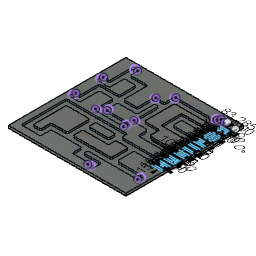
maze-v14 (Autodesk Fusion 360 design; units mm, degrees)
Autodesk Fusion 360 part; units mm, degrees
sketch "Sketch1" plane through (0, 0, 0) normal (0, 0, 1) x (1, 0, 0)
  line L0 (0, 0) -> (1000, 0)
  line L1 (1000, 0) -> (1000, 1000)
  line L2 (1000, 1000) -> (0, 1000)
  line L3 (0, 1000) -> (0, 0)
  dimension "d1" = 1000
  dimension "d2" = 1000
  constraint horizontal L0
  constraint vertical L1
  constraint horizontal L2
  constraint vertical L3
  constraint coincident L0.start L3.end
  measures "d1" distance of L0.start L2.end
  measures "d2" distance of L0.start L0.end
extrude "Extrude1" add sketch "Sketch1" along normal blind 21
sketch "top" plane through (0, 0, 21) normal (0, 0, 1) x (-1, 0, 0)
  line L0 (0, -1000) -> (0, 0)
  line L1 (0, 0) -> (-1000, 0)
  line L2 (-1000, 0) -> (-1000, -1000)
  line L3 (-1000, -1000) -> (0, -1000)
  arc A0 (-525, -126.8622) -> (-535, -116.8622) centre (-535, -126.8622) ccw
  arc A1 (-559.9586, -282.9891) -> (-569.9586, -292.9891) centre (-559.9586, -292.9891) ccw
  arc A2 (-535, -150) -> (-525, -140) centre (-535, -140) ccw
  line L4 (-300, -620.3885) -> (-300, -540)
  line L5 (-525, -140) -> (-525, -126.8622)
  arc A3 (-519.9586, -383.45) -> (-509.9586, -393.45) centre (-509.9586, -383.45) ccw
  arc A4 (-360, -282.9891) -> (-350, -272.9891) centre (-360, -272.9891) ccw
  arc A5 (-475, -140) -> (-465, -150) centre (-465, -140) ccw
  arc A6 (-579.9586, -344.6286) -> (-569.9586, -334.6286) centre (-579.9586, -334.6286) ccw
  line L6 (-569.9586, -404.6286) -> (-569.9586, -433.45)
  line L7 (-300, -332.9891) -> (-300, -383.45)
  line L8 (-300, -210) -> (-300, -283.8474)
  arc A7 (-360, -393.45) -> (-350, -383.45) centre (-360, -383.45) ccw
  arc A8 (-300, -383.45) -> (-290, -393.45) centre (-290, -383.45) ccw
  line L9 (-569.9586, -292.9891) -> (-569.9586, -334.6286)
  line L10 (-509.9586, -332.9891) -> (-360, -332.9891)
  line L11 (-519.9586, -383.45) -> (-519.9586, -342.9891)
  line L12 (-475, -200) -> (-360, -200)
  line L13 (-350, -210) -> (-350, -272.9891)
  line L14 (-890, -344.6286) -> (-735, -344.6286)
  arc A9 (-92.3471, -692.4262) -> (-82.3471, -682.4262) centre (-92.3471, -682.4262) ccw
  arc A10 (-660, -824.2821) -> (-650, -814.2821) centre (-660, -814.2821) ccw
  line L15 (-677.1097, -535) -> (-677.1097, -599.6568)
  line L16 (-700, -764.2821) -> (-700, -709.2787)
  arc A11 (-150, -897.4685) -> (-160, -887.4685) centre (-160, -897.4685) ccw
  line L17 (-300, -690.3885) -> (-300, -877.4685)
  arc A12 (-625, -56.8622) -> (-615, -66.8622) centre (-615, -56.8622) ccw
  arc A13 (-300, -877.4685) -> (-290, -887.4685) centre (-290, -877.4685) ccw
  arc A14 (-700, -709.2787) -> (-710, -699.2787) centre (-710, -709.2787) ccw
  line L18 (-132.3471, -632.4262) -> (-132.3471, -485.0006)
  line L19 (-840, -394.6286) -> (-715.6967, -394.6286)
  line L20 (-415.2274, -820.725) -> (-415.2274, -690.3885)
  arc A15 (-710, -774.2821) -> (-700, -764.2821) centre (-710, -764.2821) ccw
  line L21 (-465.2274, -770.725) -> (-465.2274, -640.3885)
  line L22 (-82.3471, -682.4262) -> (-82.3471, -525)
  arc A16 (-840, -824.2821) -> (-850, -834.2821) centre (-840, -834.2821) ccw
  line L23 (-250, -632.4262) -> (-250, -490)
  line L24 (-850, -639.2787) -> (-850, -535)
  line L25 (-497.671, -569.6568) -> (-497.671, -770.725)
  line L26 (-100, -837.4685) -> (-100, -770)
  arc A17 (-650, -659.2787) -> (-660, -649.2787) centre (-660, -659.2787) ccw
  arc A18 (-160, -837.4685) -> (-150, -827.4685) centre (-160, -827.4685) ccw
  line L27 (-290, -887.4685) -> (-160, -887.4685)
  arc A19 (-250, -632.4262) -> (-240, -642.4262) centre (-240, -632.4262) ccw
  arc A20 (-677.1097, -599.6568) -> (-667.1097, -609.6568) centre (-667.1097, -599.6568) ccw
  line L28 (-675, -334.6286) -> (-675, -210)
  line L29 (-900, -940) -> (-900, -784.2821)
  arc A21 (-627.1097, -549.6568) -> (-617.1097, -559.6568) centre (-617.1097, -549.6568) ccw
  arc A22 (-890, -774.2821) -> (-900, -784.2821) centre (-890, -784.2821) ccw
  line L30 (-715.6967, -394.6286) -> (-579.9586, -394.6286)
  arc A23 (-850, -465) -> (-840, -475) centre (-840, -465) ccw
  line L31 (-625, -50) -> (-625, -56.8622)
  line L32 (-240, -642.4262) -> (-142.3471, -642.4262)
  line L33 (-100, -837.4685) -> (-100, -950)
  arc A24 (-405.2274, -680.3885) -> (-415.2274, -690.3885) centre (-405.2274, -690.3885) ccw
  arc A25 (-725, -210) -> (-735, -200) centre (-735, -210) ccw
  line L34 (-650, -814.2821) -> (-650, -659.2787)
  line L35 (-547.671, -830.725) -> (-547.671, -857.0303)
  arc A26 (-475.2274, -780.725) -> (-465.2274, -770.725) centre (-475.2274, -770.725) ccw
  arc A27 (-677.1097, -535) -> (-687.1097, -525) centre (-687.1097, -535) ccw
  arc A28 (-140, -710.014) -> (-150, -720.014) centre (-140, -720.014) ccw
  arc A29 (-240, -692.4262) -> (-250, -702.4262) centre (-240, -702.4262) ccw
  line L36 (-650, -774.2821) -> (-649.9827, -774.2821)
  arc A30 (-675, -106.8622) -> (-665, -116.8622) centre (-665, -106.8622) ccw
  line L37 (-487.671, -830.725) -> (-425.2274, -830.725)
  line L38 (-547.671, -619.6568) -> (-547.671, -830.725)
  arc A31 (-455.2274, -630.3885) -> (-465.2274, -640.3885) centre (-455.2274, -640.3885) ccw
  line L39 (-497.671, -840.725) -> (-497.671, -907.0303)
  line L40 (-890, -774.2821) -> (-710, -774.2821)
  arc A32 (-840, -394.6286) -> (-850, -404.6286) centre (-840, -404.6286) ccw
  arc A33 (-675, -334.6286) -> (-665, -344.6286) centre (-665, -334.6286) ccw
  arc A34 (-840, -525) -> (-850, -535) centre (-840, -535) ccw
  line L41 (-627.1097, -485) -> (-627.1097, -549.6568)
  line L42 (-725, -334.6286) -> (-725, -210)
  line L43 (-675, -106.8622) -> (-675, -50)
  line L44 (-840, -475) -> (-637.1097, -475)
  line L45 (-850, -940) -> (-850, -927.0303)
  line L46 (-850, -857.0303) -> (-850, -834.2821)
  line L47 (-665, -344.6286) -> (-579.9586, -344.6286)
  line L48 (-900, -689.2787) -> (-900, -475)
  arc A35 (-735, -344.6286) -> (-725, -334.6286) centre (-735, -334.6286) ccw
  line L49 (-840, -525) -> (-687.1097, -525)
  line L50 (-840, -824.2821) -> (-660, -824.2821)
  line L51 (-675, -150) -> (-950, -150)
  line L52 (-660, -649.2787) -> (-840, -649.2787)
  arc A36 (-665, -200) -> (-675, -210) centre (-665, -210) ccw
  arc A37 (-900, -689.2787) -> (-890, -699.2787) centre (-890, -689.2787) ccw
  arc A38 (-142.3471, -642.4262) -> (-132.3471, -632.4262) centre (-142.3471, -632.4262) ccw
  arc A39 (-627.1097, -485) -> (-637.1097, -475) centre (-637.1097, -485) ccw
  line L53 (-710, -699.2787) -> (-890, -699.2787)
  arc A40 (-850, -639.2787) -> (-840, -649.2787) centre (-840, -639.2787) ccw
  arc A41 (-850, -857.0303) -> (-840, -867.0303) centre (-840, -857.0303) ccw
  arc A42 (-475, -76.8622) -> (-485, -66.8622) centre (-485, -76.8622) ccw
  line L54 (-350, -342.9891) -> (-350, -383.45)
  arc A43 (-569.9586, -433.45) -> (-559.9586, -443.45) centre (-559.9586, -433.45) ccw
  line L55 (-360, -393.45) -> (-509.9586, -393.45)
  line L56 (-300, -332.9891) -> (-300, -283.8474)
  line L57 (-465, -150) -> (-300, -150)
  arc A44 (-350, -342.9891) -> (-360, -332.9891) centre (-360, -342.9891) ccw
  line L58 (-500, -530) -> (-310, -530)
  arc A45 (-509.9586, -332.9891) -> (-519.9586, -342.9891) centre (-509.9586, -342.9891) ccw
  arc A46 (-350, -210) -> (-360, -200) centre (-360, -210) ccw
  line L59 (-360, -282.9891) -> (-559.9586, -282.9891)
  line L60 (-475, -76.8622) -> (-475, -140)
  arc A47 (-290, -200) -> (-300, -210) centre (-290, -210) ccw
  line L61 (-154.4283, -108.8474) -> (-110, -108.8474)
  arc A48 (-204.4283, -58.8474) -> (-214.4283, -68.8474) centre (-204.4283, -68.8474) ccw
  line L62 (-214.4283, -140) -> (-214.4283, -68.8474)
  arc A49 (-60, -443.45) -> (-50, -433.45) centre (-60, -433.45) ccw
  arc A50 (-110, -393.45) -> (-100, -383.45) centre (-110, -383.45) ccw
  arc A51 (-224.4283, -150) -> (-214.4283, -140) centre (-224.4283, -140) ccw
  line L63 (-164.4283, -190) -> (-164.4283, -118.8474)
  line L64 (-557.671, -867.0303) -> (-840, -867.0303)
  arc A52 (-100, -118.8474) -> (-110, -108.8474) centre (-110, -118.8474) ccw
  arc A53 (-154.4283, -108.8474) -> (-164.4283, -118.8474) centre (-154.4283, -118.8474) ccw
  arc A54 (-122.3471, -475.0006) -> (-132.3471, -485.0006) centre (-122.3471, -485.0006) ccw
  arc A55 (-174.4283, -200) -> (-164.4283, -190) centre (-174.4283, -190) ccw
  line L65 (-50, -68.8474) -> (-50, -316.2628)
  arc A56 (-50, -68.8474) -> (-60, -58.8474) centre (-60, -68.8474) ccw
  line L66 (-50, -316.2628) -> (-50, -433.45)
  line L67 (-204.4283, -58.8474) -> (-60, -58.8474)
  line L68 (-100, -118.8474) -> (-100, -383.45)
  line L69 (-617.1097, -559.6568) -> (-507.671, -559.6568)
  line L70 (-507.671, -917.0303) -> (-840, -917.0303)
  line L71 (-615, -66.8622) -> (-485, -66.8622)
  arc A57 (-569.9586, -404.6286) -> (-579.9586, -394.6286) centre (-579.9586, -404.6286) ccw
  line L72 (-140, -710.014) -> (-49.1705, -710.014)
  line L73 (-535, -116.8622) -> (-665, -116.8622)
  line L74 (-500, -480) -> (-260, -480)
  line L75 (-110, -393.45) -> (-290, -393.45)
  line L76 (-300, -150) -> (-224.4283, -150)
  line L77 (-240, -692.4262) -> (-92.3471, -692.4262)
  line L78 (-290, -200) -> (-174.4283, -200)
  line L79 (-60, -443.45) -> (-559.9586, -443.45)
  line L80 (-675, -150) -> (-535, -150)
  line L81 (-667.1097, -609.6568) -> (-557.671, -609.6568)
  arc A58 (-300, -690.3885) -> (-310, -680.3885) centre (-310, -690.3885) ccw
  line L82 (0, 0) -> (-1000, 0)
  arc A59 (-557.671, -867.0303) -> (-547.671, -857.0303) centre (-557.671, -857.0303) ccw
  line L83 (-850, -465) -> (-850, -404.6286)
  arc A60 (-310, -630.3885) -> (-300, -620.3885) centre (-310, -620.3885) ccw
  arc A61 (-497.671, -770.725) -> (-487.671, -780.725) centre (-487.671, -770.725) ccw
  line L84 (-250, -702.4262) -> (-250, -827.4685)
  line L85 (-665, -200) -> (-475, -200)
  line L86 (-405.2274, -680.3885) -> (-310, -680.3885)
  line L87 (-1000, 0) -> (-1000, -1000)
  line L88 (-900, -475) -> (-900, -354.6286)
  line L89 (-150, -897.4685) -> (-150, -950)
  line L90 (-150, -827.4685) -> (-150, -720.014)
  line L91 (-1000, -1000) -> (0, -1000)
  line L92 (-455.2274, -630.3885) -> (-310, -630.3885)
  arc A62 (-487.671, -830.725) -> (-497.671, -840.725) centre (-487.671, -840.725) ccw
  line L93 (-240, -837.4685) -> (-160, -837.4685)
  line L94 (-487.671, -780.725) -> (-475.2274, -780.725)
  line L95 (-0.0099, -1000) -> (-0.0018, 0)
  arc A63 (-250, -827.4685) -> (-240, -837.4685) centre (-240, -827.4685) ccw
  arc A64 (-890, -344.6286) -> (-900, -354.6286) centre (-890, -354.6286) ccw
  line L96 (-90, -760) -> (-50.0078, -760)
  arc A65 (-90, -760) -> (-100, -770) centre (-90, -770) ccw
  line L97 (-735, -200) -> (-950, -200)
  line L98 (-122.3471, -475.0006) -> (-49.8349, -475.0006)
  line L99 (-0.0056, -475.0006) -> (0, -475.0006)
  line L100 (-82.3471, -525) -> (-50.0058, -525)
  line L101 (-860, -950) -> (-890, -950)
  arc A66 (-250, -490) -> (-260, -480) centre (-260, -490) ccw
  arc A67 (-300, -540) -> (-310, -530) centre (-310, -540) ccw
  arc A68 (-425.2274, -830.725) -> (-415.2274, -820.725) centre (-425.2274, -820.725) ccw
  arc A69 (-497.671, -569.6568) -> (-507.671, -559.6568) centre (-507.671, -569.6568) ccw
  arc A70 (-547.671, -619.6568) -> (-557.671, -609.6568) centre (-557.671, -619.6568) ccw
  arc A71 (-507.671, -917.0303) -> (-497.671, -907.0303) centre (-507.671, -907.0303) ccw
  arc A72 (-840, -917.0303) -> (-850, -927.0303) centre (-840, -927.0303) ccw
  arc A73 (-860, -950) -> (-850, -940) centre (-860, -940) ccw
  arc A74 (-900, -940) -> (-890, -950) centre (-890, -940) ccw
  arc A75 (-950, -150) -> (-950, -200) centre (-950, -175) ccw
  arc A76 (-625, -50) -> (-675, -50) centre (-650, -50) ccw
  arc A77 (-50.0058, -525) -> (-50.1768, -475.0006) centre (-50.0058, -500) ccw
  arc A78 (-50.0078, -760) -> (-50.845, -710.014) centre (-50.0078, -735) ccw
  arc A79 (-150, -950) -> (-100, -950) centre (-125, -950) ccw
  arc A80 (-500, -480) -> (-500, -530) centre (-500, -505) ccw
  point P0 (-1000, -1000)
  dimension "d67" = 50
  dimension "d68" = 50
  dimension "d69" = 90
  dimension "d70" = 50
  dimension "d71" = 50
  dimension "d72" = 50
  dimension "d73" = 50
  dimension "d74" = 50
  dimension "d75" = 50
  dimension "d76" = 50
  dimension "d77" = 50
  dimension "d78" = 50
  dimension "d79" = 50
  dimension "d81" = 50
  dimension "d83" = 50
  dimension "d84" = 50
  dimension "d85" = 50
  dimension "d86" = 50
  dimension "d87" = 50
  dimension "d88" = 50
  dimension "d89" = 50
  dimension "d90" = 50
  dimension "d91" = 50
  dimension "d93" = 50
  dimension "d94" = 50
  dimension "d95" = 50
  dimension "d96" = 50
  dimension "d97" = 50
  dimension "d98" = 50
  dimension "d99" = 50
  dimension "d100" = 50
  dimension "d101" = 50
  dimension "d102" = 50
  dimension "d103" = 50
  dimension "d104" = 50
  dimension "d105" = 50
  dimension "d106" = 50
  dimension "d107" = 10
  dimension "d108" = 10
  dimension "d109" = 50
  dimension "d110" = 10
  dimension "d111" = 50
  dimension "d112" = 50
  dimension "d113" = 50
  dimension "d114" = 50
  dimension "d115" = 50
  dimension "d116" = 50
  dimension "d117" = 50
  dimension "d118" = 50
  dimension "d119" = 50
  dimension "d120" = 50
  dimension "d123" = 10
  dimension "d125" = 90
  dimension "d126" = 10
  dimension "d128" = 90
  dimension "d131" = 50
  dimension "d185" = 10
  dimension "d186" = 10
  constraint vertical L45
  constraint perpendicular L45 L50
  constraint perpendicular L34 L50
  constraint perpendicular L34 L52
  constraint perpendicular L24 L52
  constraint perpendicular L24 L49
  constraint perpendicular L15 L49
  constraint perpendicular L15 L81
  constraint perpendicular L38 L81
  constraint perpendicular L15 L37
  constraint perpendicular L20 L81
  constraint perpendicular L20 L86
  constraint perpendicular L23 L86
  constraint vertical L29
  constraint perpendicular L16 L53
  constraint coincident L36.start L34
  constraint collinear L36 L40
  constraint perpendicular L48 L53
  constraint perpendicular L44 L48
  constraint perpendicular L41 L53
  constraint perpendicular L41 L69
  constraint perpendicular L25 L69
  constraint perpendicular L41 L94
  constraint perpendicular L21 L69
  constraint perpendicular L41 L92
  constraint perpendicular L4 L92
  constraint tangent L58 A80
  constraint perpendicular L4 L58
  constraint tangent L74 A80
  constraint horizontal L74
  constraint perpendicular L44 L88
  constraint perpendicular L14 L88
  constraint perpendicular L14 L42
  constraint perpendicular L44 L83
  constraint perpendicular L19 L24
  constraint perpendicular L28 L44
  constraint perpendicular L24 L51
  constraint perpendicular L84 L86
  constraint perpendicular L84 L93
  constraint perpendicular L33 L86
  constraint perpendicular L17 L86
  constraint perpendicular L17 L27
  constraint perpendicular L27 L89
  constraint perpendicular L23 L32
  constraint perpendicular L18 L32
  constraint perpendicular L23 L77
  constraint perpendicular L22 L77
  constraint perpendicular L18 L98
  constraint perpendicular L26 L93
  constraint perpendicular L90 L93
  constraint perpendicular L72 L90
  constraint perpendicular L37 L39
  constraint perpendicular L45 L70
  constraint perpendicular L35 L37
  constraint perpendicular L45 L64
  constraint perpendicular L28 L80
  constraint perpendicular L5 L80
  constraint perpendicular L28 L73
  constraint perpendicular L43 L73
  constraint perpendicular L31 L73
  constraint perpendicular L31 L71
  constraint perpendicular L28 L85
  constraint perpendicular L57 L60
  constraint perpendicular L8 L57
  constraint perpendicular L12 L60
  constraint perpendicular L12 L13
  constraint perpendicular L13 L59
  constraint perpendicular L9 L12
  constraint perpendicular L10 L11
  constraint perpendicular L10 L56
  constraint perpendicular L8 L76
  constraint perpendicular L57 L62
  constraint perpendicular L62 L67
  constraint perpendicular L57 L65
  constraint perpendicular L8 L78
  constraint perpendicular L63 L78
  constraint perpendicular L61 L63
  constraint perpendicular L61 L68
  constraint vertical L68
  constraint parallel L65 L66
  constraint perpendicular L68 L75
  constraint perpendicular L66 L79
  constraint vertical L11
  constraint collinear L45 L46
  constraint perpendicular L54 L75
  constraint perpendicular L7 L75
  constraint collinear L55 L75
  constraint perpendicular L9 L47
  constraint perpendicular L9 L30
  constraint collinear L6 L9
  constraint tangent A12 L31
  constraint tangent A12 L71
  constraint tangent A30 L73
  constraint tangent A30 L43
  constraint equal A12 A30
  constraint tangent A0 L5
  constraint tangent A0 L73
  constraint equal A0 A12
  constraint tangent A42 L71
  constraint tangent A42 L60
  constraint tangent A5 L57
  constraint tangent A5 L60
  constraint equal A5 A42
  constraint tangent A2 L80
  constraint tangent A2 L5
  constraint equal A2 A42
  constraint tangent A36 L85
  constraint tangent L28 A36
  constraint tangent A25 L42
  constraint equal A25 A36
  constraint tangent L14 A35
  constraint tangent L42 A35
  constraint equal A35 A36
  constraint tangent A33 L47
  constraint tangent L28 A33
  constraint equal A33 A36
  constraint tangent A32 L83
  constraint tangent L19 A32
  constraint equal A32 A36
  constraint tangent A23 L83
  constraint tangent A23 L44
  constraint equal A23 A36
  constraint tangent L44 A39
  constraint tangent L41 A39
  constraint equal A36 A39
  constraint tangent A21 L41
  constraint tangent A21 L69
  constraint equal A21 A36
  constraint tangent A27 L49
  constraint tangent L15 A27
  constraint equal A27 A36
  constraint tangent L15 A20
  constraint tangent A20 L81
  constraint equal A20 A36
  constraint tangent L24 A34
  constraint tangent A34 L49
  constraint equal A34 A36
  constraint tangent L52 A40
  constraint tangent L24 A40
  constraint equal A36 A40
  constraint tangent A37 L53
  constraint tangent L48 A37
  constraint equal A36 A37
  constraint tangent A17 L34
  constraint tangent A17 L52
  constraint equal A17 A36
  constraint tangent L16 A14
  constraint tangent A14 L53
  constraint equal A14 A36
  constraint tangent L16 A15
  constraint tangent A15 L40
  constraint equal A15 A36
  constraint tangent A16 L50
  constraint tangent A16 L46
  constraint equal A16 A36
  constraint tangent L29 A22
  constraint tangent A22 L40
  constraint equal A22 A36
  constraint tangent A41 L64
  constraint tangent L46 A41
  constraint equal A36 A41
  constraint tangent L35 A59
  constraint tangent L64 A59
  constraint equal A36 A59
  constraint tangent L39 A62
  constraint tangent L37 A62
  constraint equal A36 A62
  constraint tangent L25 A61
  constraint tangent A61 L94
  constraint equal A36 A61
  constraint tangent A26 L94
  constraint tangent L21 A26
  constraint equal A26 A36
  constraint tangent L20 A24
  constraint tangent A24 L86
  constraint equal A24 A36
  constraint tangent L21 A31
  constraint tangent A31 L92
  constraint equal A31 A36
  constraint tangent L17 A58
  constraint tangent A58 L86
  constraint equal A36 A58
  constraint tangent A60 L92
  constraint tangent L4 A60
  constraint equal A36 A60
  constraint tangent A19 L32
  constraint tangent L23 A19
  constraint equal A19 A36
  constraint tangent A29 L84
  constraint tangent A29 L77
  constraint equal A29 A36
  constraint tangent A9 L77
  constraint tangent A9 L22
  constraint equal A9 A36
  constraint tangent L32 A38
  constraint tangent L18 A38
  constraint equal A36 A38
  constraint tangent L84 A63
  constraint tangent L93 A63
  constraint equal A36 A63
  constraint tangent L17 A13
  constraint tangent A13 L27
  constraint equal A13 A36
  constraint tangent A18 L90
  constraint tangent A18 L93
  constraint equal A18 A36
  constraint tangent A11 L27
  constraint tangent A11 L89
  constraint equal A11 A36
  constraint tangent A28 L90
  constraint tangent A28 L72
  constraint equal A28 A36
  constraint tangent L18 A54
  constraint tangent A54 L98
  constraint equal A36 A54
  constraint tangent A49 L66
  constraint tangent A49 L79
  constraint equal A36 A49
  constraint tangent A50 L68
  constraint tangent A50 L75
  constraint equal A36 A50
  constraint tangent L7 A8
  constraint tangent A8 L75
  constraint equal A8 A36
  constraint tangent A7 L54
  constraint tangent A7 L55
  constraint equal A7 A36
  constraint tangent L54 A44
  constraint tangent L10 A44
  constraint equal A36 A44
  constraint tangent A4 L13
  constraint tangent A4 L59
  constraint equal A4 A36
  constraint tangent L12 A46
  constraint tangent L13 A46
  constraint equal A36 A46
  constraint tangent A47 L78
  constraint tangent L8 A47
  constraint equal A36 A47
  constraint tangent A55 L78
  constraint tangent L63 A55
  constraint equal A36 A55
  constraint tangent L63 A53
  constraint tangent L61 A53
  constraint equal A36 A53
  constraint tangent A48 L62
  constraint tangent A48 L67
  constraint equal A36 A48
  constraint tangent L61 A52
  constraint tangent A52 L68
  constraint equal A36 A52
  constraint tangent A56 L67
  constraint tangent L65 A56
  constraint equal A36 A56
  constraint tangent L11 A45
  constraint tangent L10 A45
  constraint equal A36 A45
  constraint tangent A3 L11
  constraint tangent A3 L55
  constraint equal A3 A36
  constraint tangent L30 A57
  constraint tangent L6 A57
  constraint equal A36 A57
  constraint tangent A43 L79
  constraint tangent L6 A43
  constraint equal A36 A43
  constraint tangent A6 L47
  constraint tangent A6 L9
  constraint equal A6 A36
  constraint tangent A1 L59
  constraint tangent A1 L9
  constraint equal A1 A36
  constraint tangent A51 L76
  constraint tangent L62 A51
  constraint equal A36 A51
  constraint tangent A10 L50
  constraint tangent A10 L34
  constraint equal A10 A36
  constraint tangent L14 A64
  constraint tangent L88 A64
  constraint coincident L72.end A78
  constraint tangent L96 A78
  constraint tangent L26 A65
  constraint tangent L96 A65
  constraint tangent L97 A75
  constraint perpendicular L28 L97
  constraint perpendicular L29 L91
  constraint coincident L98.end A77
  constraint coincident L95 L99.start
  constraint collinear L98 L99
  constraint tangent L100 A77
  constraint perpendicular L29 L101
  constraint tangent L23 A66
  constraint tangent L74 A66
  constraint tangent L4 A67
  constraint tangent L58 A67
  constraint equal A66 A67
  constraint tangent L20 A68
  constraint tangent L37 A68
  constraint equal A66 A68
  constraint tangent L25 A69
  constraint tangent L69 A69
  constraint tangent L38 A70
  constraint tangent L81 A70
  constraint equal A69 A70
  constraint tangent L39 A71
  constraint tangent L70 A71
  constraint equal A69 A71
  constraint tangent L45 A72
  constraint tangent L70 A72
  constraint equal A69 A72
  constraint tangent L101 A73
  constraint tangent L45 A73
  constraint equal A69 A73
  constraint tangent L101 A74
  constraint tangent L29 A74
  constraint equal A69 A74
  constraint coincident L98 A77.end
  constraint coincident L72 A78.end
  measures "d67" diameter of A80
  measures "d68" distance of L29 L45
  measures "d69" angle of L29 L40
  measures "d70" distance of L64 L70
  measures "d71" distance of L25 L38
  measures "d72" distance of L35 L39
  measures "d73" distance of L37 L94
  measures "d74" distance of L20 L21
  measures "d75" distance of L86 L92
  measures "d76" distance of L32 L77
  measures "d77" distance of L17 L84
  measures "d78" distance of L27 L93
  measures "d79" distance of L26 L90
  measures "d81" distance of L18 L22
  measures "d83" distance of L69 L81
  measures "d84" distance of L15 L41
  measures "d85" distance of L44 L49
  measures "d86" distance of L40 L50
  measures "d87" distance of L16 L34
  measures "d88" distance of L52 L53
  measures "d89" distance of L24 L48
  measures "d90" distance of L14 L19
  measures "d91" distance of L28 L42
  measures "d93" distance of L12 L57
  measures "d94" distance of L76 L78
  measures "d95" distance of L5 L60
  measures "d96" distance of L71 L73
  measures "d97" distance of L31 L43
  measures "d98" distance of L62 L63
  measures "d99" distance of L61 L67
  measures "d100" distance of L65 L68
  measures "d101" distance of L75 L79
  measures "d102" distance of L9 L11
  measures "d103" distance of L10 L59
  measures "d104" distance of L8 L13
  measures "d105" distance of L7 L54
  measures "d106" distance of L30 L47
  measures "d107" radius of A12
  measures "d108" radius of A42
  measures "d109" distance of L80 L85
  measures "d110" radius of A36
  measures "d111" diameter of A79
  measures "d112" diameter of A78
  measures "d113" distance of A78.centre L95
  measures "d114" distance of A79.centre L91
  measures "d115" diameter of A77
  measures "d116" distance of A77.centre L95
  measures "d117" diameter of A76
  measures "d118" distance of A76.centre L82
  measures "d119" diameter of A75
  measures "d120" distance of A75.centre L87
  measures "d123" radius of A64
  measures "d125" angle of L26 L96
  measures "d126" radius of A65
  measures "d128" angle of L22 L100
  measures "d131" distance of L91 L101
  measures "d185" radius of A66
  measures "d186" radius of A69
extrude "Extrude3" cut sketch "top" against normal blind 15 contours A0 A2 L4 L5 A5 L6 L14 A9 L16 A11 L17 A12 A13 A14 L18 L19 L20 A15 L21 L22 L23 L25 L26 A18 L27 A19 L29 A21 A22 L30 A23 L31 L32 L33 A24 A25 A26 A28 A29 A30 L37 A31 L39 L40 A32 L41 L42 L43 L44 L45 L48 A35 L51 A37 A38 A39 L53 A42 A43 L57 L58 L60 A48 L62 A49 A51 A54 L65 A56 L66 L67 L69 L70 L71 A57 L72 L73 L74 L76 L77 L79 L80 A58 L83 A60 A61 L84 L86 L88 L89 L90 L92 A62 L93 L94 A63 A64 L96 A65 L97 L98 L100 L101 A66 A67 A68 A69 A71 A72 A73 A74 A75 A76 A77 A78 A79 A80
sketch "Sketch4" plane through (0, 0, 21) normal (0, 0, 1) x (-1, 0, 0)
  line L0 (0, -1000) -> (0, 0)
  line L1 (0, 0) -> (-1000, 0)
  line L2 (-1000, 0) -> (-1000, -1000)
  line L3 (-1000, -1000) -> (0, -1000)
  line L4 (-625, -50) -> (-625, -56.8622)
  arc A0 (-625, -56.8622) -> (-615, -66.8622) centre (-615, -56.8622) ccw
  line L5 (-615, -66.8622) -> (-485, -66.8622)
  arc A1 (-475, -76.8622) -> (-485, -66.8622) centre (-485, -76.8622) ccw
  line L6 (-475, -76.8622) -> (-475, -140)
  arc A2 (-475, -140) -> (-465, -150) centre (-465, -140) ccw
  line L7 (-465, -150) -> (-224.4283, -150)
  arc A3 (-224.4283, -150) -> (-214.4283, -140) centre (-224.4283, -140) ccw
  line L8 (-214.4283, -140) -> (-214.4283, -68.8474)
  arc A4 (-204.4283, -58.8474) -> (-214.4283, -68.8474) centre (-204.4283, -68.8474) ccw
  line L9 (-204.4283, -58.8474) -> (-60, -58.8474)
  arc A5 (-50, -68.8474) -> (-60, -58.8474) centre (-60, -68.8474) ccw
  line L10 (-50, -68.8474) -> (-50, -433.45)
  arc A6 (-60, -443.45) -> (-50, -433.45) centre (-60, -433.45) ccw
  line L11 (-60, -443.45) -> (-559.9586, -443.45)
  arc A7 (-569.9586, -433.45) -> (-559.9586, -443.45) centre (-559.9586, -433.45) ccw
  line L12 (-569.9586, -433.45) -> (-569.9586, -404.6286)
  arc A8 (-569.9586, -404.6286) -> (-579.9586, -394.6286) centre (-579.9586, -404.6286) ccw
  line L13 (-579.9586, -394.6286) -> (-840, -394.6286)
  arc A9 (-840, -394.6286) -> (-850, -404.6286) centre (-840, -404.6286) ccw
  line L14 (-850, -404.6286) -> (-850, -465)
  arc A10 (-850, -465) -> (-840, -475) centre (-840, -465) ccw
  line L15 (-840, -475) -> (-637.1097, -475)
  arc A11 (-627.1097, -485) -> (-637.1097, -475) centre (-637.1097, -485) ccw
  line L16 (-627.1097, -485) -> (-627.1097, -549.6568)
  arc A12 (-627.1097, -549.6568) -> (-617.1097, -559.6568) centre (-617.1097, -549.6568) ccw
  line L17 (-617.1097, -559.6568) -> (-507.671, -559.6568)
  line L18 (-497.671, -569.6568) -> (-497.671, -770.725)
  arc A13 (-497.671, -770.725) -> (-487.671, -780.725) centre (-487.671, -770.725) ccw
  line L19 (-487.671, -780.725) -> (-475.2274, -780.725)
  arc A14 (-475.2274, -780.725) -> (-465.2274, -770.725) centre (-475.2274, -770.725) ccw
  line L20 (-465.2274, -770.725) -> (-465.2274, -640.3885)
  arc A15 (-455.2274, -630.3885) -> (-465.2274, -640.3885) centre (-455.2274, -640.3885) ccw
  line L21 (-455.2274, -630.3885) -> (-310, -630.3885)
  arc A16 (-310, -630.3885) -> (-300, -620.3885) centre (-310, -620.3885) ccw
  line L22 (-300, -620.3885) -> (-300, -540)
  line L23 (-310, -530) -> (-500, -530)
  line L24 (-500, -480) -> (-260, -480)
  line L25 (-250, -490) -> (-250, -632.4262)
  arc A17 (-250, -632.4262) -> (-240, -642.4262) centre (-240, -632.4262) ccw
  line L26 (-240, -642.4262) -> (-142.3471, -642.4262)
  arc A18 (-142.3471, -642.4262) -> (-132.3471, -632.4262) centre (-142.3471, -632.4262) ccw
  line L27 (-132.3471, -632.4262) -> (-132.3471, -485.0006)
  arc A19 (-122.3471, -475.0006) -> (-132.3471, -485.0006) centre (-122.3471, -485.0006) ccw
  line L28 (-122.3471, -475.0006) -> (-49.8349, -475.0006)
  line L29 (-50.0058, -525) -> (-82.3471, -525)
  line L30 (-82.3471, -525) -> (-82.3471, -682.4262)
  arc A20 (-92.3471, -692.4262) -> (-82.3471, -682.4262) centre (-92.3471, -682.4262) ccw
  line L31 (-92.3471, -692.4262) -> (-240, -692.4262)
  arc A21 (-240, -692.4262) -> (-250, -702.4262) centre (-240, -702.4262) ccw
  line L32 (-250, -702.4262) -> (-250, -827.4685)
  arc A22 (-250, -827.4685) -> (-240, -837.4685) centre (-240, -827.4685) ccw
  line L33 (-240, -837.4685) -> (-160, -837.4685)
  arc A23 (-160, -837.4685) -> (-150, -827.4685) centre (-160, -827.4685) ccw
  line L34 (-150, -827.4685) -> (-150, -720.014)
  arc A24 (-140, -710.014) -> (-150, -720.014) centre (-140, -720.014) ccw
  line L35 (-140, -710.014) -> (-49.1705, -710.014)
  line L36 (-50.0078, -760) -> (-90, -760)
  arc A25 (-90, -760) -> (-100, -770) centre (-90, -770) ccw
  line L37 (-100, -770) -> (-100, -950)
  line L38 (-150, -950) -> (-150, -897.4685)
  arc A26 (-150, -897.4685) -> (-160, -887.4685) centre (-160, -897.4685) ccw
  line L39 (-160, -887.4685) -> (-290, -887.4685)
  arc A27 (-300, -877.4685) -> (-290, -887.4685) centre (-290, -877.4685) ccw
  line L40 (-300, -877.4685) -> (-300, -690.3885)
  arc A28 (-300, -690.3885) -> (-310, -680.3885) centre (-310, -690.3885) ccw
  line L41 (-310, -680.3885) -> (-405.2274, -680.3885)
  arc A29 (-405.2274, -680.3885) -> (-415.2274, -690.3885) centre (-405.2274, -690.3885) ccw
  line L42 (-415.2274, -690.3885) -> (-415.2274, -820.725)
  line L43 (-425.2274, -830.725) -> (-487.671, -830.725)
  arc A30 (-487.671, -830.725) -> (-497.671, -840.725) centre (-487.671, -840.725) ccw
  line L44 (-497.671, -840.725) -> (-497.671, -907.0303)
  line L45 (-507.671, -917.0303) -> (-840, -917.0303)
  line L46 (-850, -927.0303) -> (-850, -940)
  line L47 (-860, -950) -> (-890, -950)
  line L48 (-900, -940) -> (-900, -784.2821)
  arc A31 (-890, -774.2821) -> (-900, -784.2821) centre (-890, -784.2821) ccw
  line L49 (-890, -774.2821) -> (-710, -774.2821)
  arc A32 (-710, -774.2821) -> (-700, -764.2821) centre (-710, -764.2821) ccw
  line L50 (-700, -764.2821) -> (-700, -709.2787)
  arc A33 (-700, -709.2787) -> (-710, -699.2787) centre (-710, -709.2787) ccw
  line L51 (-710, -699.2787) -> (-890, -699.2787)
  arc A34 (-900, -689.2787) -> (-890, -699.2787) centre (-890, -689.2787) ccw
  line L52 (-900, -689.2787) -> (-900, -354.6286)
  arc A35 (-890, -344.6286) -> (-900, -354.6286) centre (-890, -354.6286) ccw
  line L53 (-890, -344.6286) -> (-735, -344.6286)
  arc A36 (-735, -344.6286) -> (-725, -334.6286) centre (-735, -334.6286) ccw
  line L54 (-725, -334.6286) -> (-725, -210)
  arc A37 (-725, -210) -> (-735, -200) centre (-735, -210) ccw
  line L55 (-735, -200) -> (-950, -200)
  line L56 (-950, -150) -> (-535, -150)
  arc A38 (-535, -150) -> (-525, -140) centre (-535, -140) ccw
  line L57 (-525, -140) -> (-525, -126.8622)
  arc A39 (-525, -126.8622) -> (-535, -116.8622) centre (-535, -126.8622) ccw
  line L58 (-535, -116.8622) -> (-665, -116.8622)
  arc A40 (-675, -106.8622) -> (-665, -116.8622) centre (-665, -106.8622) ccw
  line L59 (-675, -106.8622) -> (-675, -50)
  line L60 (-925, -369.5248) -> (-925, -329.1557)
  line L61 (-925, -329.1557) -> (-978.2852, -329.1557)
  line L62 (-978.2852, -329.1557) -> (-978.2852, -369.5248)
  line L63 (-978.2852, -369.5248) -> (-960.4047, -369.5248)
  line L64 (-960.4047, -369.5248) -> (-960.4047, -353.081)
  line L65 (-925, -369.5248) -> (-939.7027, -369.5248)
  line L66 (-960.4047, -353.081) -> (-945.4047, -353.081)
  line L67 (-945.4047, -353.081) -> (-945.4047, -384.5248)
  line L68 (-945.4047, -384.5248) -> (-993.2852, -384.5248)
  line L69 (-993.2852, -384.5248) -> (-993.2852, -314.1557)
  line L70 (-993.2852, -314.1557) -> (-910, -314.1557)
  line L71 (-910, -314.1557) -> (-910, -384.5248)
  line L72 (-910, -384.5248) -> (-939.7027, -384.5248)
  line L73 (-939.7027, -369.5248) -> (-939.7027, -384.5248)
  line L74 (-993.2852, -384.5248) -> (-993.2852, -940) construction
  line L75 (-910, -384.5248) -> (-910, -955.0751) construction
  line L76 (-910, -414.5248) -> (-993.2852, -414.5248)
  line L77 (-910, -414.5248) -> (-910, -464.4098)
  line L78 (-976.2029, -464.4098) -> (-976.2029, -443.949)
  line L79 (-976.2029, -443.949) -> (-993.2852, -470.6982)
  line L80 (-976.2029, -464.4098) -> (-910, -464.4098)
  line L81 (-993.2852, -470.6982) -> (-993.2852, -442.8287)
  line L82 (-984.7891, -429.5248) -> (-993.2852, -429.5248)
  line L83 (-925, -429.5248) -> (-961.2029, -429.5248)
  line L84 (-961.2029, -429.5248) -> (-961.2029, -449.4098)
  line L85 (-961.2029, -449.4098) -> (-925, -449.4098)
  line L86 (-925, -449.4098) -> (-925, -429.5248)
  line L87 (-910, -500.6982) -> (-993.2852, -500.6982)
  line L88 (-993.2852, -500.6982) -> (-993.2852, -544.5165)
  line L89 (-993.2852, -544.5165) -> (-910, -544.5165)
  line L90 (-910, -544.5165) -> (-910, -500.6982)
  line L91 (-925, -515.6982) -> (-978.2852, -515.6982)
  line L92 (-978.2852, -515.6982) -> (-978.2852, -529.5165)
  line L93 (-978.2852, -529.5165) -> (-925, -529.5165)
  line L94 (-925, -529.5165) -> (-925, -515.6982)
  line L95 (-910, -574.5165) -> (-993.2852, -574.5165)
  line L96 (-993.2852, -574.5165) -> (-993.2852, -638.3566)
  line L97 (-910, -638.3566) -> (-993.2852, -638.3566)
  line L98 (-910, -623.3566) -> (-978.2852, -623.3566)
  line L99 (-978.2852, -623.3566) -> (-978.2852, -589.5165)
  line L100 (-978.2852, -589.5165) -> (-910, -589.5165)
  line L101 (-910, -574.5165) -> (-910, -589.5165)
  line L102 (-910, -623.3566) -> (-910, -638.3566)
  line L103 (-910, -668.3566) -> (-993.2852, -668.3566)
  line L104 (-993.2852, -683.3566) -> (-953.9977, -683.3566)
  line L105 (-953.9977, -683.3566) -> (-953.9977, -714.3075)
  line L106 (-953.9977, -714.3075) -> (-910, -714.3075)
  line L107 (-993.2852, -683.3566) -> (-993.2852, -668.3566)
  line L108 (-910, -668.3566) -> (-910, -714.3075)
  line L109 (-925, -683.3566) -> (-938.9977, -683.3566)
  line L110 (-938.9977, -683.3566) -> (-938.9977, -699.3075)
  line L111 (-938.9977, -699.3075) -> (-925, -699.3075)
  line L112 (-925, -699.3075) -> (-925, -683.3566)
  line L113 (-993.2852, -759.3075) -> (-993.2852, -774.3075)
  line L114 (-910, -774.3075) -> (-910, -759.3075)
  line L115 (-993.2852, -789.3075) -> (-993.2852, -804.3075)
  line L116 (-910, -804.3075) -> (-910, -789.3075)
  line L117 (-940, -819.3075) -> (-925, -819.3075)
  line L118 (-978.2852, -819.3075) -> (-963.2852, -819.3075)
  line L119 (-963.2852, -744.3075) -> (-978.2852, -744.3075)
  line L120 (-978.2852, -897.3011) -> (-910, -897.3011)
  line L121 (-910, -877.7997) -> (-930.1428, -854.2428)
  line L122 (-930.1428, -854.2428) -> (-941.5433, -863.991)
  line L123 (-941.5433, -863.991) -> (-925.8869, -882.3011)
  line L124 (-925.8869, -882.3011) -> (-978.2852, -882.3011)
  line L125 (-978.2852, -882.3011) -> (-978.2852, -860.7687)
  line L126 (-978.2852, -860.7687) -> (-993.2852, -860.7687)
  line L127 (-978.2852, -921.978) -> (-993.2852, -921.978)
  line L128 (-910, -877.7997) -> (-910, -897.3011)
  line L129 (-963.2852, -759.3075) -> (-963.2852, -744.3075)
  line L130 (-978.2852, -759.3075) -> (-993.2852, -759.3075)
  line L131 (-993.2852, -774.3075) -> (-978.2852, -774.3075)
  line L132 (-978.2852, -744.3075) -> (-978.2852, -759.3075)
  line L133 (-978.2852, -774.3075) -> (-978.2852, -789.3075)
  line L134 (-978.2852, -804.3075) -> (-978.2852, -819.3075)
  line L135 (-963.2852, -819.3075) -> (-963.2852, -804.3075)
  line L136 (-963.2852, -789.3075) -> (-963.2852, -774.3075)
  line L137 (-978.2852, -789.3075) -> (-993.2852, -789.3075)
  line L138 (-993.2852, -804.3075) -> (-978.2852, -804.3075)
  line L139 (-940, -804.3075) -> (-940, -819.3075)
  line L140 (-925, -819.3075) -> (-925, -804.3075)
  line L141 (-963.2852, -804.3075) -> (-940, -804.3075)
  line L142 (-925, -804.3075) -> (-910, -804.3075)
  line L143 (-910, -789.3075) -> (-925, -789.3075)
  line L144 (-940, -789.3075) -> (-963.2852, -789.3075)
  line L145 (-963.2852, -774.3075) -> (-940, -774.3075)
  line L146 (-925, -774.3075) -> (-910, -774.3075)
  line L147 (-910, -759.3075) -> (-925, -759.3075)
  line L148 (-940, -759.3075) -> (-963.2852, -759.3075)
  line L149 (-940, -744.3075) -> (-940, -759.3075)
  line L150 (-940, -774.3075) -> (-940, -789.3075)
  line L151 (-925, -789.3075) -> (-925, -774.3075)
  line L152 (-925, -759.3075) -> (-925, -744.3075)
  line L153 (-925, -744.3075) -> (-940, -744.3075)
  line L154 (-993.2852, -429.5248) -> (-993.2852, -414.5248)
  line L155 (-984.7891, -429.5248) -> (-993.2852, -442.8287)
  line L156 (-978.2852, -921.978) -> (-978.2852, -897.3011)
  line L157 (-993.2852, -860.7687) -> (-993.2852, -921.978)
  arc A41 (-300, -540) -> (-310, -530) centre (-310, -540) ccw
  arc A42 (-250, -490) -> (-260, -480) centre (-260, -490) ccw
  arc A43 (-425.2274, -830.725) -> (-415.2274, -820.725) centre (-425.2274, -820.725) ccw
  arc A44 (-497.671, -569.6568) -> (-507.671, -559.6568) centre (-507.671, -569.6568) ccw
  arc A45 (-507.671, -917.0303) -> (-497.671, -907.0303) centre (-507.671, -907.0303) ccw
  arc A46 (-840, -917.0303) -> (-850, -927.0303) centre (-840, -927.0303) ccw
  arc A47 (-860, -950) -> (-850, -940) centre (-860, -940) ccw
  arc A48 (-900, -940) -> (-890, -950) centre (-890, -940) ccw
  arc A49 (-50.0058, -525) -> (-49.8349, -475.0006) centre (-50.0058, -500) ccw
  arc A50 (-50.0078, -760) -> (-49.1705, -710.014) centre (-50.0078, -735) ccw
  arc A51 (-150, -950) -> (-100, -950) centre (-125, -950) ccw
  arc A52 (-950, -150) -> (-950, -200) centre (-950, -175) ccw
  arc A53 (-625, -50) -> (-675, -50) centre (-650, -50) ccw
  arc A54 (-500, -480) -> (-500, -530) centre (-500, -505) ccw
  dimension "d132" = 90
  dimension "d135" = 15
  dimension "d137" = 15
  dimension "d138" = 15
  dimension "d139" = 15
  dimension "d140" = 15
  dimension "d141" = 15
  dimension "d142" = 15
  dimension "d143" = 15
  dimension "d144" = 15
  dimension "d145" = 15
  dimension "d146" = 30
  dimension "d147" = 30
  dimension "d148" = 30
  dimension "d149" = 30
  dimension "d150" = 30
  dimension "d151" = 15
  dimension "d152" = 15
  dimension "d153" = 15
  dimension "d154" = 15
  dimension "d155" = 15
  dimension "d156" = 15
  dimension "d157" = 15
  dimension "d158" = 15
  dimension "d159" = 15
  dimension "d160" = 15
  dimension "d162" = 15
  dimension "d163" = 15
  dimension "d164" = 15
  dimension "d165" = 15
  dimension "d166" = 15
  dimension "d167" = 15
  dimension "d168" = 15
  dimension "d169" = 15
  dimension "d170" = 15
  dimension "d171" = 15
  dimension "d172" = 15
  dimension "d173" = 15
  dimension "d174" = 15
  dimension "d175" = 15
  dimension "d176" = 15
  dimension "d177" = 15
  dimension "d178" = 83.2852
  dimension "d179" = 15
  dimension "d181" = 10
  dimension "d254" = 15
  constraint perpendicular L53 L60
  constraint perpendicular L60 L61
  constraint perpendicular L53 L62
  constraint perpendicular L62 L63
  constraint perpendicular L63 L64
  constraint perpendicular L60 L65
  constraint perpendicular L64 L66
  constraint perpendicular L66 L67
  constraint perpendicular L64 L68
  constraint perpendicular L68 L69
  constraint perpendicular L69 L70
  constraint perpendicular L68 L71
  constraint perpendicular L69 L72
  constraint vertical L73
  constraint perpendicular L68 L74
  constraint perpendicular L72 L75
  constraint coincident L75 L76.start
  constraint coincident L74 L76.end
  constraint perpendicular L74 L76
  constraint coincident L75 L77.end
  constraint perpendicular L76 L78
  constraint coincident L74 L79.end
  constraint perpendicular L75 L80
  constraint coincident L74 L81.end
  constraint coincident L74 L82.end
  constraint horizontal L83
  constraint vertical L84
  constraint horizontal L85
  constraint vertical L86
  constraint horizontal L87
  constraint vertical L88
  constraint horizontal L89
  constraint vertical L90
  constraint coincident L74 L88.end
  constraint coincident L75 L87.start
  constraint horizontal L91
  constraint vertical L92
  constraint horizontal L93
  constraint vertical L94
  constraint coincident L75 L95.start
  constraint coincident L74 L95.end
  constraint perpendicular L74 L95
  constraint coincident L74 L96.end
  constraint coincident L75 L97.start
  constraint perpendicular L96 L97
  constraint coincident L75 L98.start
  constraint perpendicular L75 L98
  constraint perpendicular L98 L99
  constraint coincident L75 L100.end
  constraint perpendicular L75 L100
  constraint coincident L75 L103.start
  constraint coincident L74 L103.end
  constraint perpendicular L74 L103
  constraint coincident L74 L104.start
  constraint perpendicular L74 L104
  constraint perpendicular L104 L105
  constraint coincident L75 L106.end
  constraint perpendicular L75 L106
  constraint horizontal L109
  constraint vertical L110
  constraint horizontal L111
  constraint vertical L112
  constraint horizontal L147
  constraint vertical L113
  constraint horizontal L131
  constraint vertical L114
  constraint coincident L74 L113.end
  constraint coincident L75 L114.end
  constraint horizontal L143
  constraint vertical L115
  constraint horizontal L138
  constraint vertical L116
  constraint coincident L74 L115.end
  constraint coincident L75 L116.end
  constraint vertical L149
  constraint horizontal L117
  constraint vertical L140
  constraint horizontal L118
  constraint vertical L135
  constraint horizontal L119
  constraint vertical L132
  constraint coincident L74 L127.end
  constraint coincident L75 L120.end
  constraint perpendicular L75 L120
  constraint coincident L75 L121.start
  constraint perpendicular L121 L122
  constraint perpendicular L122 L123
  constraint perpendicular L75 L124
  constraint perpendicular L124 L125
  constraint coincident L136.end L131
  constraint collinear L129 L135
  constraint collinear L130 L147
  constraint coincident L131.end L132
  constraint collinear L131 L145
  constraint collinear L132 L133
  constraint coincident L133.end L143
  constraint collinear L133 L134
  constraint coincident L135.end L138
  constraint collinear L135 L136
  constraint collinear L137 L143
  constraint collinear L138 L141
  constraint coincident L144.start L143
  constraint collinear L139 L149
  constraint coincident L140.end L141
  constraint collinear L140 L151
  constraint collinear L141 L142
  constraint collinear L143 L144
  constraint coincident L145.end L149
  constraint collinear L145 L146
  constraint coincident L147.end L151
  constraint collinear L147 L148
  constraint collinear L149 L150
  constraint collinear L151 L152
  constraint perpendicular L149 L153
  constraint collinear L68 L72
  constraint horizontal L82
  constraint parallel L79 L155
  constraint coincident L74 L126.end
  constraint perpendicular L120 L156
  constraint perpendicular L127 L157
  measures "d132" angle of L125 L126
  measures "d135" distance of L145 L148
  measures "d137" distance of L133 L136
  measures "d138" distance of L141 L144
  measures "d139" distance of L150 L151
  measures "d140" distance of L75 L151
  measures "d141" distance of L74 L133
  measures "d142" distance of L117.end L140.end
  measures "d143" distance of L152.end L147.end
  measures "d144" distance of L119.start L129.start
  measures "d145" distance of L118.start L134.start
  measures "d146" distance of L68 L76
  measures "d147" distance of L79.end L87.end
  measures "d148" distance of L88.end L95.end
  measures "d149" distance of L96.end L103.end
  measures "d150" distance of L106 L153
  measures "d151" distance of L61 L70
  measures "d152" distance of L62 L69
  measures "d153" distance of L63 L68
  measures "d154" distance of L64 L67
  measures "d155" distance of L65 L72
  measures "d156" distance of L60 L71
  measures "d157" distance of L77 L86
  measures "d158" distance of L80 L85
  measures "d159" distance of L78 L84
  measures "d160" distance of L76 L83
  measures "d162" distance of L76 L82
  measures "d163" distance of L79 L155
  measures "d164" distance of L87 L91
  measures "d165" distance of L89 L93
  measures "d166" distance of L88 L92
  measures "d167" distance of L90 L94
  measures "d168" distance of L95 L100
  measures "d169" distance of L96 L99
  measures "d170" distance of L97 L98
  measures "d171" distance of L103 L104
  measures "d172" distance of L105 L110
  measures "d173" distance of L106 L111
  measures "d174" distance of L108 L112
  measures "d175" distance of L103 L109
  measures "d176" distance of L121 L123
  measures "d177" distance of L120 L124
  measures "d178" distance of L74 L75
  measures "d179" distance of L156 L157
  measures "d181" distance of L52 L75
  measures "d254" distance of L144 L145
extrude "Extrude4" [suppressed]
sketch "vcarve" plane through (0, 0, 0) normal (0, 0, 1) x (1, 0, 0)
equation "þykkt_maze = 50 mm"
equation "horn_maze = 10 mm"
equation "base = 50 mm"
equation "maze = 15 mm"
equation "d67 = þykkt_maze"
equation "d68 = þykkt_maze"
equation "d70 = þykkt_maze"
equation "d71 = þykkt_maze"
equation "d72 = þykkt_maze"
equation "d73 = þykkt_maze"
equation "d74 = þykkt_maze"
equation "d75 = þykkt_maze"
equation "d76 = þykkt_maze"
equation "d77 = þykkt_maze"
equation "d78 = þykkt_maze"
equation "d79 = þykkt_maze"
equation "d81 = þykkt_maze"
equation "d83 = þykkt_maze"
equation "d84 = þykkt_maze"
equation "d85 = þykkt_maze"
equation "d86 = þykkt_maze"
equation "d87 = þykkt_maze"
equation "d88 = þykkt_maze"
equation "d89 = þykkt_maze"
equation "d90 = þykkt_maze"
equation "d91 = þykkt_maze"
equation "d93 = þykkt_maze"
equation "d94 = þykkt_maze"
equation "d95 = þykkt_maze"
equation "d96 = þykkt_maze"
equation "d97 = þykkt_maze"
equation "d98 = þykkt_maze"
equation "d99 = þykkt_maze"
equation "d100 = þykkt_maze"
equation "d101 = þykkt_maze"
equation "d102 = þykkt_maze"
equation "d103 = þykkt_maze"
equation "d104 = þykkt_maze"
equation "d105 = þykkt_maze"
equation "d106 = þykkt_maze"
equation "d107 = horn_maze"
equation "d108 = horn_maze"
equation "d109 = þykkt_maze"
equation "d110 = horn_maze"
equation "d111 = þykkt_maze"
equation "d112 = þykkt_maze"
equation "d113 = þykkt_maze"
equation "d114 = þykkt_maze"
equation "d115 = þykkt_maze"
equation "d116 = þykkt_maze"
equation "d117 = þykkt_maze"
equation "d118 = þykkt_maze"
equation "d119 = þykkt_maze"
equation "d120 = þykkt_maze"
equation "d123 = horn_maze"
equation "d129 = -maze"
equation "d131 = þykkt_maze"
equation "carving = 5 mm"
equation "brennimerki = 5 mm"
equation "d183 = -brennimerki"
equation "d185 = horn_maze"
equation "d186 = horn_maze"
